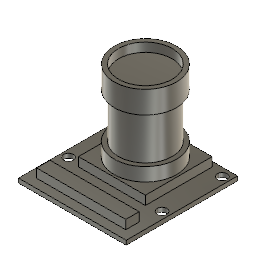
DualCamFixture (Autodesk Fusion 360 archive; units mm, degrees)
design "Camera"
Autodesk Fusion 360 part; units mm, degrees
sketch "Sketch1" plane through (0, 0, 0) normal (0, 0, -1) x (1, 0, 0)
  circle A0 centre (10.5, -6.75) radius 1.1
  circle A1 centre (-10.5, -6.75) radius 1.1
  circle A2 centre (10.5, 6.75) radius 1.1
  circle A3 centre (-10.5, 6.75) radius 1.1
  line L0 (12.1, -8.6) -> (12.1, 16.4)
  line L1 (12.1, 16.4) -> (-12.1, 16.4)
  line L2 (-12.1, 16.4) -> (-12.1, -8.6)
  line L3 (-12.1, -8.6) -> (12.1, -8.6)
  line L4 (10, 14.4) -> (-10, 14.4)
  line L5 (-10, 14.4) -> (-10, 11.4)
  line L6 (-10, 11.4) -> (10, 11.4)
  line L7 (10, 11.4) -> (10, 14.4)
  line L8 (10, 14.4) -> (-10, 11.4) construction
  line L9 (-10, 14.4) -> (10, 11.4) construction
  circle A4 centre (0, 0) radius 6
  circle A5 centre (0, 0) radius 7
  line L10 (7.5, 7.5) -> (-7.5, 7.5)
  line L11 (-7.5, 7.5) -> (-7.5, -7.5)
  line L12 (-7.5, -7.5) -> (7.5, -7.5)
  line L13 (7.5, -7.5) -> (7.5, 7.5)
  line L14 (7.5, 7.5) -> (-7.5, -7.5) construction
  line L15 (-7.5, 7.5) -> (7.5, -7.5) construction
  point P0 (0, 12.9)
  dimension "d1" = 20
  dimension "d2" = 3
  dimension "d3" = 15
  dimension "d4" = 15
  dimension "d5" = 12
  dimension "d6" = 14
  dimension "d7" = 2
  constraint horizontal L4
  constraint perpendicular L4 L5
  constraint parallel L4 L6
  constraint parallel L5 L7
  constraint coincident L8 P0
  constraint coincident L9 P0
  constraint coincident A4.centre A5.centre
  constraint concentric A4 A5
  constraint horizontal L10
  constraint perpendicular L10 L11
  constraint parallel L10 L12
  constraint parallel L11 L13
  constraint coincident L14 A4.centre
  constraint coincident L15 A4.centre
  constraint vertical P0 A4.centre
  measures "d1" distance of L5.end L6.end
  measures "d2" distance of L4.end L5.end
  measures "d3" distance of L11.end L12.end
  measures "d4" distance of L10.end L11.end
  measures "d5" diameter of A4
  measures "d6" diameter of A5
  measures "d7" distance of L1 L4
extrude "Extrude3" add sketch "Sketch1" against normal blind 1 contours L0 L1 L2 L3
extrude "Extrude4" add sketch "Sketch1" against normal blind 3 contours L4 L5 L6 L7
extrude "Extrude5" add sketch "Sketch1" against normal blind 3 contours L10 L11 L12 L13
extrude "Extrude6" add sketch "Sketch1" against normal blind 6 contours A5
extrude "Extrude7" add sketch "Sketch1" against normal blind 19 contours A4
extrude "Extrude8" add sketch "Sketch1" against normal blind 5 from surface at -16 contours A5
